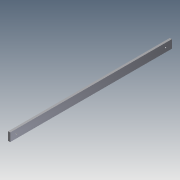
# Autodesk Inventor part: it (tech) support
Saved by Autodesk Inventor 2011 (Build 150239000, 239)
## iProperties
Created: 2011-12-03
Part Number: it (tech) support
Document SubType Name: Modeling
Designer: Matthew
Density: 1 g/cm^3
Author: Matthew
Autodesk Inventor part; units mm, degrees
ref_plane "YZ Plane" through (0, 0, 0) normal (1, 0, 0) x (0, 1, 0)
ref_plane "XZ Plane" through (0, 0, 0) normal (0, 1, 0) x (-1, 0, 0)
ref_plane "XY Plane" through (0, 0, 0) normal (0, 0, 1) x (1, 0, 0)
sketch "Sketch1" plane through (0, 0, 0) normal (0, 0, 1) x (1, 0, 0)
  line L0 (-3.0179, 9.9103) -> (3.3321, 9.9103)
  line L1 (3.3321, 9.9103) -> (3.3321, -15.4897)
  line L2 (3.3321, -15.4897) -> (-3.0179, -15.4897)
  line L3 (-3.0179, -15.4897) -> (-3.0179, 9.9103)
  point P0 (0, 0)
  dimension "d0" = 6.35
  dimension "d1" = 25.4
  constraints: 8 end point, 2 parallel, 1 horizontal, 1 perpendicular
  measures "d0" distance of L1.end L2.end
  measures "d1" distance of L0.end L1.end
extrude "Extrusion1" add sketch "Sketch1" along normal blind 495.3
sketch "Sketch2" plane through (-3.0179, -15.4897, 0) normal (-1, 0, 0) x (0, 0, 1)
  line L0 (0, 25.4) -> (495.3, 25.4) projected
  line L1 (0, 0) -> (0, 25.4) projected
  line L2 (0, 0) -> (495.3, 0) projected
  line L3 (495.3, 25.4) -> (463.55, 25.4)
  line L4 (495.3, 0) -> (488.95, 0)
  line L5 (488.95, 0) -> (463.55, 25.4)
  line L6 (488.95, 25.4) -> (463.55, 0)
  circle A0 centre (476.25, 12.7) radius 1.9812
  line L7 (0, 12.7) -> (60.7, 12.7)
  line L8 (0, 0) -> (31.75, 0)
  line L9 (31.75, 0) -> (9.4445, 22.3055)
  circle A1 centre (19.05, 12.7) radius 1.9818
  point P0 (0, 15.4897)
  dimension "d4" = 31.75
  dimension "d5" = 6.35
  dimension "d6" = 3.9624
  dimension "d7" = 31.75
  dimension "d8" = 45
  constraints: 14 end point, 7 point on line, 2 centre point, 2 midpoint, 1 parallel, 1 perpendicular
  measures "d4" distance of L0.end L3.end
  measures "d5" distance of L2.end L4.end
  measures "d6" diameter of A0
  measures "d7" distance of L1.start L8.end
  measures "d8" angle of L9 L8
extrude "Extrusion2" cut sketch "Sketch2" against normal blind 25.4 contours A0 L6 L5 | L5 L6 A0 | A1 L9 L7 | L7 L9 A1 | A0 L5 L6 | L5 A0 L6 | L9 A1 L7 | L7 A1 L9
body "Solid1"
